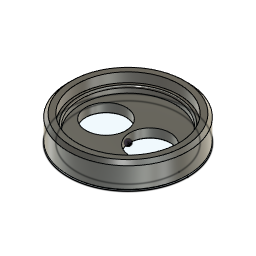
_Double 32mm Magnet Base W_ Step.f6e80f6f-a3bb-4c85-a733-1b3eea0858f7 (Autodesk Fusion 360 design; units mm, degrees)
Autodesk Fusion 360 part; units mm, degrees
note: some values were not read from the file. Chosen so that the rebuilt part matches the saved one: which face or edge a step refers to; that a step has no effect. Set by a fixed rule: which sketch regions a step uses.
sketch "Sketch1" plane through (0, 0, 0) normal (0, 0, 1) x (1, 0, 0)
  circle A0 centre (0, 0) radius 16.25
  circle A1 centre (0, 0) radius 19
  dimension "d1" = 32.5
  dimension "d2" = 38
  constraint coincident A0.centre A1.centre
  constraint concentric A0 A1
  measures "d1" diameter of A0
  measures "d2" diameter of A1
extrude "Extrude1" add sketch "Sketch1" along normal blind 8
extrude "Extrude2" add sketch "Sketch1" along normal blind 3 contours A0
chamfer "Chamfer1" distance 1 angle 45 1 edges at (-17.7142, -6.8707, 8)
chamfer "Chamfer2" [no effect]
sketch "Sketch2" plane through (0, 0, 3) normal (0, 0, 1) x (-1, 0, 0)
  circle A0 centre (0, 0) radius 16.25
  circle A1 centre (0, 0) radius 15
  dimension "d10" = 30
  constraint coincident A0.centre A1.centre
  measures "d10" diameter of A1
extrude "Extrude3" add sketch "Sketch2" along normal blind 2
fillet "Fillet1" radius 0.5 1 edges at (13.9849, -5.4242, 5)
chamfer "Chamfer3" distance 0.5 angle 45 1 edges at (-17.7142, -6.8707, 0)
sketch "Sketch3" plane through (0, 0, 0) normal (0, 0, 1) x (1, 0, 0)
move_face "OffsetFaces1" [no effect]
sketch "Sketch4" plane through (0, 0, 0) normal (0, 0, 1) x (1, 0, 0)
  circle A0 centre (-7, 0) radius 6.4
  circle A1 centre (7, 0) radius 6.4
  dimension "d17" = 12.8
  dimension "d18" = 12.8
  measures "d17" diameter of A0
  measures "d18" diameter of A1
extrude "Extrude4" cut sketch "Sketch4" along normal blind 4
chamfer "Chamfer4" distance 0.25 angle 45 1 edges at (-12.9669, -2.3143, 0)
chamfer "Chamfer5" distance 0.25 angle 45 1 edges at (1.0331, -2.3143, 0)
